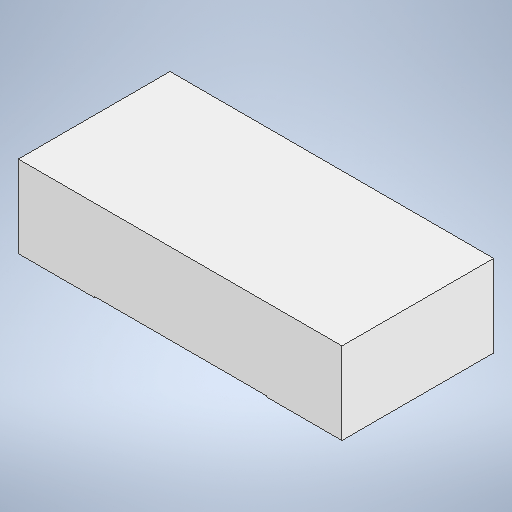
# Autodesk Inventor part: 32kHz-crystal
Saved by Autodesk Inventor 2025.2 (Build 292293000, 293)
## iProperties
Created: 2024-12-27
Part Number: 32kHz-crystal
Material: Generic
Document SubType Name: Modeling
Designer: tyson
Density: 1 g/cm^3
Appearance: Default
Author: tyson
Autodesk Inventor part; units mm, degrees
ref_plane "YZ Plane" through (0, 0, 0) normal (1, 0, 0) x (0, 1, 0)
ref_plane "XZ Plane" through (0, 0, 0) normal (0, 1, 0) x (-1, 0, 0)
ref_plane "XY Plane" through (0, 0, 0) normal (0, 0, 1) x (1, 0, 0)
sketch "Sketch1" plane through (0, 0, 0) normal (0, 1, 0) x (-1, 0, 0)
  line L0 (1.6, -0.75) -> (-1.6, -0.75)
  line L1 (-1.6, -0.75) -> (-1.6, 0.75)
  line L2 (-1.6, 0.75) -> (1.6, 0.75)
  line L3 (1.6, 0.75) -> (1.6, -0.75)
  line L4 (1.6, -0.75) -> (-1.6, 0.75) construction
  line L5 (-1.6, -0.75) -> (1.6, 0.75) construction
  point P0 (0, 0)
  dimension "d2" = 3.2
  dimension "d3" = 1.5
  constraints: 12 end point, 2 midpoint, 2 parallel, 1 horizontal, 1 perpendicular
  measures "d2" distance of L0.start L0.end
  measures "d3" distance of L0.end L1.end
extrude "Extrusion1" add sketch "Sketch1" along normal blind 0.8
sketch "Sketch2" plane through (0, 0, 0) normal (0, -1, 0) x (1, 0, 0)
  line L0 (1.6, 0.75) -> (1.6, -0.75) projected
  line L1 (1.6, 0.75) -> (0.85, 0.75)
  line L2 (0.85, 0.75) -> (0.85, -0.5)
  line L3 (1.1, -0.75) -> (1.6, -0.75)
  line L4 (1.6, -0.75) -> (1.6, 0.75)
  circle A0 centre (0.85, -0.75) radius 0.25 construction
  line L5 (1.1, -0.75) -> (0.85, -0.5)
  point P0 (0, 0)
  dimension "d7" = 0.5
  dimension "d8" = 0.75
  constraints: 10 end point, 2 parallel, 2 point on circle, 1 centre point, 1 horizontal, 1 perpendicular
  measures "d7" diameter of A0
  measures "d8" distance of L0.start L1.end
extrude "Extrusion2" add sketch "Sketch2" along normal blind 0.01
sketch "Sketch3" plane through (0, 0, 0) normal (0, -1, 0) x (1, 0, 0)
  line L0 (-1.6, 0.75) -> (1.6, 0.75) projected
  line L1 (-1.6, 0.75) -> (-0.85, 0.75)
  line L2 (-0.85, 0.75) -> (-0.85, -0.75)
  line L3 (-0.85, -0.75) -> (-1.6, -0.75)
  line L4 (-1.6, -0.75) -> (-1.6, 0.75)
  point P0 (0, 0)
  dimension "d11" = 0.75
  dimension "d12" = 1.5
  constraints: 8 end point, 2 parallel, 1 horizontal, 1 perpendicular
  measures "d11" distance of L2.end L3.end
  measures "d12" distance of L1.end L2.end
extrude "Extrusion3" add sketch "Sketch3" along normal blind 0.01
body "Solid1"
